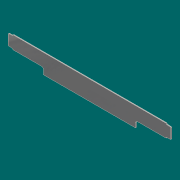
# Autodesk Inventor part: A1-18002-100-40 Pocket door plate
Saved by Autodesk Inventor 2017 (Build 210142000, 142)
## iProperties
Created: 2018-01-26
Part Number: A1-18002-100-40 Pocket door plate
Material: Steel, Mild
Document SubType Name: Modeling
Designer: Graeme_Van_Dongen
Density: 7.85 g/cm^3
Appearance: Steel
Mass: 7280.19 g
Surface Area: 3089.76 cm^2
Volume: 927.412 cm^3
Description: 47 3/8" x 5 5/8" x 1/4" PLATE, 44W
Author: Graeme_Van_Dongen
Autodesk Inventor part; units mm, degrees
ref_plane "YZ Plane" through (0, 0, 0) normal (1, 0, 0) x (0, 1, 0)
ref_plane "XZ Plane" through (0, 0, 0) normal (0, 1, 0) x (-1, 0, 0)
ref_plane "XY Plane" through (0, 0, 0) normal (0, 0, 1) x (1, 0, 0)
sketch "Sketch1" plane through (0, 0, 0) normal (0, 0, 1) x (1, 0, 0)
  line L0 (-339.725, 0) -> (339.725, 0)
  line L1 (339.725, 0) -> (339.725, 47.625)
  line L2 (339.725, 47.625) -> (566.1025, 47.625)
  line L3 (601.6625, 59.2709) -> (601.6625, 131.2291)
  line L4 (566.1025, 142.875) -> (-566.1025, 142.875)
  line L5 (-601.6625, 131.2291) -> (-601.6625, 59.2709)
  line L6 (-566.1025, 47.625) -> (-339.725, 47.625)
  line L7 (-339.725, 47.625) -> (-339.725, 0)
  line L8 (566.1025, 47.625) -> (566.1025, 48.9204)
  arc A0 (571.2291, 54.3232) -> (566.1025, 48.9204) centre (571.5127, 48.9204) ccw
  line L9 (571.2291, 54.3232) -> (598.317, 55.7452)
  arc A1 (598.317, 55.7452) -> (601.6625, 59.2709) centre (598.1319, 59.2709) ccw
  line L10 (566.1025, 142.875) -> (566.1025, 141.5796)
  arc A2 (566.1025, 141.5796) -> (571.2291, 136.1768) centre (571.5127, 141.5796) ccw
  line L11 (571.2291, 136.1768) -> (598.317, 134.7548)
  arc A3 (601.6625, 131.2291) -> (598.317, 134.7548) centre (598.1319, 131.2291) ccw
  line L12 (-566.1025, 142.875) -> (-566.1025, 141.5796)
  arc A4 (-571.2291, 136.1768) -> (-566.1025, 141.5796) centre (-571.5127, 141.5796) ccw
  line L13 (-571.2291, 136.1768) -> (-598.317, 134.7548)
  arc A5 (-598.317, 134.7548) -> (-601.6625, 131.2291) centre (-598.1319, 131.2291) ccw
  line L14 (-566.1025, 47.625) -> (-566.1025, 48.9204)
  arc A6 (-566.1025, 48.9204) -> (-571.2291, 54.3232) centre (-571.5127, 48.9204) ccw
  line L15 (-571.2291, 54.3232) -> (-598.317, 55.7452)
  arc A7 (-601.6625, 59.2709) -> (-598.317, 55.7452) centre (-598.1319, 59.2709) ccw
  point P0 (0, 0)
  point P1 (0, 0)
  dimension "d0" = 679.45
  dimension "d1" = 1203.325
  dimension "d2" = 47.625
  dimension "d3" = 95.25
  dimension "d4" = 71.9582
  dimension "d8" = 3.5306
  dimension "d9" = 5.4102
  dimension "d10" = 35.56
  dimension "d11" = 1.2954
  constraints: 32 end point, 16 point on circle, 16 tangent, 8 centre point, 7 equal length, 6 equal radius, 4 point on line, 3 perpendicular, 3 vertical, 2 collinear, 1 coincident, 1 horizontal, 1 midpoint, 1 parallel, 3 other
  measures "d0" distance of L0.start L0.end
  measures "d1" distance between parallel lines of L3 L5
  measures "d2" distance of L6.end L0.start
  measures "d3" distance between parallel lines of L4 L6
  measures "d4" distance of L5.start L5.end
  measures "d8" radius of A5
  measures "d9" radius of A4
  measures "d10" distance between parallel lines of L12 L5
  measures "d11" distance of L4.end L12.end
extrude "Extrusion1" add sketch "Sketch1" along normal blind 6.35
fillet "Fillet1" radius 15.875 2 edges at (-339.725, 47.625, 3.175) (339.725, 47.625, 3.175)
body "Solid1"
